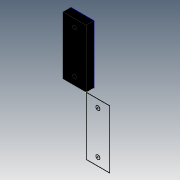
# Autodesk Inventor part: holderBlock
Saved by Autodesk Inventor 2015 (Build 190159000, 159)
## iProperties
Created: 2014-08-31
Part Number: holderBlock
Material: Generic
Document SubType Name: Modeling
Designer: shohei
Density: 1 g/cm^3
Appearance: Default
Mass: 176.858 g
Surface Area: 273.425 cm^2
Volume: 176.858 cm^3
Author: shohei
Autodesk Inventor part; units mm, degrees
ref_plane "YZ Plane" through (0, 0, 0) normal (1, 0, 0) x (0, 1, 0)
ref_plane "XZ Plane" through (0, 0, 0) normal (0, 1, 0) x (-1, 0, 0)
ref_plane "XY Plane" through (0, 0, 0) normal (0, 0, 1) x (1, 0, 0)
sketch "Block1" plane through (0, 0, 0) normal (0, 0, 1) x (1, 0, 0)
  line L0 (-60.22, 0.22) -> (-60.22, -150.22)
  line L1 (-60.22, -150.22) -> (0.22, -150.22)
  line L2 (0.22, -150.22) -> (0.22, 0.22)
  line L3 (0.22, 0.22) -> (-60.22, 0.22)
  circle A0 centre (-30, -20) radius 5.22
  circle A1 centre (-30, -130) radius 5.22
  point P0 (-30, -75)
sketch "Sketch1" plane through (0, 0, 0) normal (0, 1, 0) x (-1, 0, 0)
  line L0 (0, 0) -> (60, 0)
  line L1 (60, 0) -> (60, 150)
  line L2 (60, 150) -> (0, 150)
  line L3 (0, 150) -> (0, 0)
  circle A0 centre (30, 130) radius 5
  circle A1 centre (30, 20) radius 5
  dimension "d0" = 60
  dimension "d1" = 150
  dimension "d4" = 10
  dimension "d5" = 10
  dimension "d6" = 20
  dimension "d7" = 20
  dimension "d8" = 30
  dimension "d11" = 30
  constraints: 8 end point, 2 centre point, 2 parallel, 1 horizontal, 1 perpendicular
  measures "d0" distance of L1.end L2.end
  measures "d1" distance of L0.end L1.end
  measures "d4" diameter of A0
  measures "d5" diameter of A1
  measures "d6" distance from line of L2 A0.centre
  measures "d7" distance from line of L0 A1.centre
  measures "d8" distance from line of L3 A0.centre
  measures "d11" distance from line of L3 A1.centre
extrude "Extrusion2" add sketch "Sketch1" along normal blind 20
sketch "Sketch2" plane through (0, 20, 0) normal (0, 1, 0) x (1, 0, 0)
  line L0 (0, -150) -> (0, 0) projected
  line L1 (-60, -150) -> (0, -150) projected
  line L2 (-60, 0) -> (-60, -150) projected
  circle A0 centre (-30, -130) radius 5 projected
  circle A1 centre (-30, -20) radius 5 projected
  line L3 (0, 0) -> (-60, 0) projected
  constraints: 3 perpendicular, 2 other
sketch "DXF" plane through (0, 0, 0) normal (0, 1, 0) x (-1, 0, 0)
  point P0 (0, 0)
equation "\"d8\" = 0.5 * d0"
equation "\"d11\" = 0.5 * d0"
body "Solid2"
